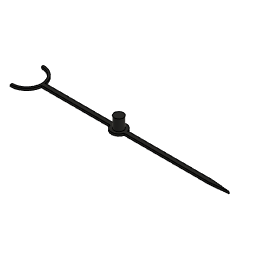
pointer (Autodesk Fusion 360 design; units mm, degrees)
Autodesk Fusion 360 part; units mm, degrees
sketch "Sketch1" plane through (0, 0, 0) normal (0, 0, 1) x (1, 0, 0)
  line L0 (-50, 1) -> (50, -1) construction
  line L1 (50, 1) -> (-50, -1) construction
  line L2 (50, 1) -> (60, 1) construction
  line L3 (50, -1) -> (60, -1) construction
  arc A0 (-50, -8) -> (-50, 8) centre (-50, 0) ccw
  line L4 (-50, 9) -> (-50, 8)
  line L5 (-50, -8) -> (-50, -9)
  line L6 (50, 1) -> (59.9497, -0.002)
  line L7 (59.9497, -0.002) -> (50, -1)
  arc A1 (3.9992, -0.08) -> (3.9992, 0.08) centre (0, 0) ccw
  arc A2 (3.873, 1) -> (-3.873, 1) centre (0, 0) ccw
  arc A3 (-3.9992, 0.08) -> (-3.9992, -0.08) centre (0, 0) ccw
  arc A4 (-3.873, -1) -> (3.873, -1) centre (0, 0) ccw
  arc A5 (-50, -9) -> (-41.0557, -1) centre (-50, 0) ccw
  arc A6 (-41.0557, 1) -> (-50, 9) centre (-50, 0) ccw
  line L8 (-41.0557, 1) -> (-3.873, 1)
  line L9 (3.873, 1) -> (50, 1)
  line L10 (50, -1) -> (3.873, -1)
  line L11 (-3.873, -1) -> (-41.0557, -1)
  dimension "d57" = 8
  dimension "d58" = 100
  dimension "d59" = 2
  dimension "d64" = 8
  dimension "d66" = 10
  constraint coincident A1.centre A2.centre
  constraint horizontal L8
  constraint parallel L8 L10
  constraint coincident L0 A1.centre
  constraint coincident L1 A1.centre
  constraint horizontal L2
  constraint horizontal L3
  constraint coincident L1 A1.end
  constraint coincident A2.start L8
  constraint coincident L0 A1.start
  constraint concentric A1 A2
  constraint coincident L0 A3.start
  constraint concentric A2 A3
  constraint coincident L1 A3.end
  constraint coincident A4.start L10
  constraint concentric A3 A4
  constraint concentric A0 A5
  constraint concentric A5 A6
  constraint collinear L8 L9
  constraint collinear L10 L11
  measures "d57" diameter of A2
  measures "d58" distance of L0.end L1.end
  measures "d59" distance of L1.start L0.end
  measures "d64" radius of A0
  measures "d66" distance of L1.start L6.end
extrude "Extrude1" add sketch "Sketch1" along normal blind 1
sketch "Sketch2" plane through (0, 0, 1) normal (0, 0, 1) x (-1, 0, 0)
  arc A0 (-3.873, -1) -> (3.873, -1) centre (0, 0) ccw
  line L0 (3.873, -1) -> (41.0557, -1)
  arc A1 (41.0557, -1) -> (50, -9) centre (50, 0) ccw
  line L1 (50, -9) -> (50, -8)
  arc A2 (50, 8) -> (50, -8) centre (50, 0) ccw
  line L2 (50, 8) -> (50, 9)
  arc A3 (50, 9) -> (41.0557, 1) centre (50, 0) ccw
  line L3 (41.0557, 1) -> (3.873, 1)
  arc A4 (3.873, 1) -> (-3.873, 1) centre (0, 0) ccw
  line L4 (-3.873, 1) -> (-50, 1)
  line L5 (-50, 1) -> (-59.9497, 0.002)
  line L6 (-59.9497, 0.002) -> (-50, -1)
  line L7 (-50, -1) -> (-3.873, -1)
  circle A5 centre (0, 0) radius 2.485
  dimension "d69" = 4.97
  constraint coincident A0.centre A4.centre
  measures "d69" diameter of A5
extrude "Extrude2" add sketch "Sketch2" along normal blind 6 contours A5
